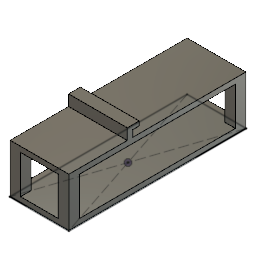
BoardRack_LEDCube_V1 (Autodesk Fusion 360 design; units mm, degrees)
Autodesk Fusion 360 part; units mm, degrees
sketch "Sketch1" plane through (0, 0, 0) normal (0, 1, 0) x (1, 0, 0)
  line L0 (-8.9, 26.75) -> (8.9, 26.75)
  line L1 (8.9, 26.75) -> (8.9, -26.75)
  line L2 (8.9, -26.75) -> (-8.9, -26.75)
  line L3 (-8.9, -26.75) -> (-8.9, 26.75)
  line L4 (-8.9, 26.75) -> (8.9, -26.75) construction
  line L5 (8.9, 26.75) -> (-8.9, -26.75) construction
  dimension "d1" = 17.8
  dimension "d2" = 53.5
  constraint perpendicular L0 L1
  constraint parallel L0 L2
  constraint parallel L1 L3
  constraint horizontal L0
  constraint coincident L4 origin
  constraint coincident L5 origin
  measures "d1" distance of L0.start L0.end
  measures "d2" distance of L0.end L1.end
extrude "Extrude4" add sketch "Sketch1" along normal blind 1.6 makes body 1
extrude "Extrude1" add sketch "Sketch1" along normal blind 1.6 separate body makes body 2
sketch "Sketch2" plane through (0, 1.6, 0) normal (0, 1, 0) x (-1, 0, 0)
  line L0 (8.9, 26.75) -> (-8.9, 26.75)
  line L1 (-8.9, 26.75) -> (-8.9, -26.75)
  line L2 (-8.9, -26.75) -> (8.9, -26.75)
  line L3 (8.9, -26.75) -> (8.9, 26.75)
  line L4 (8.9, -26.75) -> (5.7, -26.75)
  line L5 (5.7, -26.75) -> (5.7, -23.55)
  line L6 (5.7, -23.55) -> (8.9, -23.55)
  line L7 (8.9, -23.55) -> (8.9, -26.75)
  line L8 (-5.65, -26.75) -> (-8.85, -26.75)
  line L9 (-8.85, -26.75) -> (-8.85, -23.55)
  line L10 (-8.85, -23.55) -> (-5.65, -23.55)
  line L11 (-5.65, -23.55) -> (-5.65, -26.75)
  line L12 (8.9, 24.05) -> (5.7, 24.05)
  line L13 (5.7, 24.05) -> (5.7, 27.25)
  line L14 (5.7, 27.25) -> (8.9, 27.25)
  line L15 (8.9, 27.25) -> (8.9, 24.05)
  line L16 (-5.65, 24.05) -> (-8.85, 24.05)
  line L17 (-8.85, 24.05) -> (-8.85, 27.25)
  line L18 (-8.85, 27.25) -> (-5.65, 27.25)
  line L19 (-5.65, 27.25) -> (-5.65, 24.05)
  point P0 (-5.65, -26.75)
  point P1 (8.9, 24.05)
  point P2 (-5.65, 24.05)
  dimension "d7" = 3.2
  dimension "d8" = 3.2
  dimension "d11" = -14.55
  dimension "d12" = 50.8
  dimension "d13" = 38.8
  constraint horizontal L4
  constraint vertical L5
  constraint horizontal L6
  constraint vertical L7
  constraint coincident L2.end L3.start
  measures "d7" distance of L4.end L5.end
  measures "d8" distance of L5.end L6.end
sketch "Sketch4" plane through (0, 1.6, 0) normal (0, 1, 0) x (-1, 0, 0)
  line L0 (8.9, 26.75) -> (-8.9, 26.75)
  line L1 (-8.9, 26.75) -> (-8.9, -26.75)
  line L2 (-8.9, -26.75) -> (8.9, -26.75)
  line L3 (8.9, -26.75) -> (8.9, 26.75)
  line L4 (8.9, -26.75) -> (5.7, -26.75)
  line L5 (5.7, -26.75) -> (5.7, -23.55)
  line L6 (5.7, -23.55) -> (8.9, -23.55)
  line L7 (8.9, -23.55) -> (8.9, -26.75)
  line L8 (-8.9, -26.75) -> (-8.9, -23.55)
  line L9 (-8.9, -23.55) -> (-5.7, -23.55)
  line L10 (-5.7, -26.75) -> (-8.9, -26.75)
  line L11 (-5.7, -23.55) -> (-5.7, -26.75)
  line L12 (5.7, 23.55) -> (5.7, 26.75)
  line L13 (5.7, 26.75) -> (8.9, 26.75)
  line L14 (8.9, 23.55) -> (5.7, 23.55)
  line L15 (8.9, 26.75) -> (8.9, 23.55)
  line L16 (-8.9, 23.55) -> (-8.9, 26.75)
  line L17 (-8.9, 26.75) -> (-5.7, 26.75)
  line L18 (-5.7, 23.55) -> (-8.9, 23.55)
  line L19 (-5.7, 26.75) -> (-5.7, 23.55)
  point P0 (8.9, -26.75)
  point P1 (-5.7, -26.75)
  point P2 (-5.7, -26.75)
  point P3 (8.9, 23.55)
  point P4 (8.9, 23.55)
  point P5 (-5.7, 23.55)
  point P6 (-5.7, 23.55)
  dimension "d24" = 3.2
  dimension "d25" = 3.2
  dimension "d28" = -14.6
  dimension "d29" = 50.3
  constraint horizontal L4
  constraint vertical L5
  constraint horizontal L6
  constraint vertical L7
  constraint coincident P0 L2.end
  measures "d24" distance of L5 P0
  measures "d25" distance of L4.end L5.end
extrude "Extrude5" add sketch "Sketch4" along normal blind 11.575 contours L0 L3 L12 L13 L14 L15 | L0 L1 L16 L17 L18 L19 | L2 L3 L4 L5 L6 L7 | L1 L2 L8 L9 L10 L11 bodies 1 2
sketch "Sketch5" plane through (0, 13.175, 0) normal (0, 1, 0) x (-1, 0, 0)
  line L0 (8.9, -23.55) -> (5.7, -23.55)
  line L1 (5.7, -23.55) -> (5.7, -26.75)
  line L2 (5.7, -26.75) -> (8.9, -26.75)
  line L3 (8.9, -26.75) -> (8.9, -23.55)
  line L4 (8.9, -26.75) -> (-8.9, -26.75)
  line L5 (-8.9, -26.75) -> (-8.9, 26.75)
  line L6 (-8.9, 26.75) -> (8.9, 26.75)
  line L7 (8.9, 26.75) -> (8.9, -26.75)
  point P0 (-8.9, 26.75)
  constraint horizontal L4
  constraint vertical L5
  constraint horizontal L6
  constraint vertical L7
  constraint coincident P0 L5.end
  constraint coincident L2.end L3.start
extrude "Extrude6" add sketch "Sketch5" along normal blind 1.6 bodies 1
sketch "Sketch6" plane through (0, 14.775, 0) normal (0, 1, 0) x (-1, 0, 0)
  line L0 (8.9, 26.75) -> (-8.9, 26.75)
  line L1 (-8.9, 26.75) -> (-8.9, -26.75)
  line L2 (-8.9, -26.75) -> (8.9, -26.75)
  line L3 (8.9, -26.75) -> (8.9, 26.75)
  line L4 (8.9, 7.5) -> (-8.9, 7.5)
  line L5 (-8.9, 7.5) -> (-8.9, 9.1)
  line L6 (-8.9, 9.1) -> (8.9, 9.1)
  line L7 (8.9, 9.1) -> (8.9, 7.5)
  line L8 (8.9, -26.75) -> (-8.9, -26.75)
  dimension "d34" = 1.6
  dimension "d35" = 34.25
  constraint horizontal L4
  constraint vertical L5
  constraint horizontal L6
  constraint vertical L7
  constraint coincident L1 L5.end
  constraint coincident L3 L4.start
  measures "d34" distance of L4.end L5.end
  measures "d35" distance of L4 L8
extrude "Extrude7" add sketch "Sketch6" along normal blind 3.3 contours L1 L3 L4 L5 L6 L7 bodies 1
sketch "Sketch7" plane through (0, 0, 7.5) normal (0, 0, -1) x (-1, 0, 0)
  line L0 (-8.9, 14.775) -> (8.9, 14.775)
  line L1 (8.9, 14.775) -> (8.9, 18.075)
  line L2 (8.9, 18.075) -> (-8.9, 18.075)
  line L3 (-8.9, 18.075) -> (-8.9, 14.775)
  line L4 (-8.9, 18.075) -> (8.9, 18.075)
  line L5 (8.9, 18.075) -> (8.9, 16.775)
  line L6 (8.9, 16.775) -> (-8.9, 16.775)
  line L7 (-8.9, 16.775) -> (-8.9, 18.075)
  dimension "d38" = 1.3
  constraint horizontal L4
  constraint horizontal L6
  constraint coincident L2.end L3.start
  measures "d38" distance of L2.end L6.end
extrude "Extrude8" add sketch "Sketch7" along normal blind 2 contours L1 L2 L3 L4 L5 L6 L7 bodies 1
equation "d1 = boxWidth"
equation "d11 = -17.75 mm + 3.2 mm"
equation "d12 = 54 mm - 3.2 mm"
equation "BoxLength = 53.5 mm"
equation "boxWidth = 17.8 mm"
equation "d28 = -17.8 mm + 3.2 mm"
equation "d29 = 53.5 mm - 3.2 mm"
equation "d30 = 14.075 mm - 2.5 mm"
